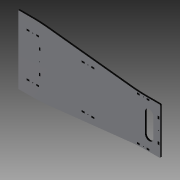
# Autodesk Inventor part: SIDE PLATE
Saved by Autodesk Inventor 2013 (Build 170138000, 138)
## iProperties
Created: 2014-06-21
Part Number: SIDE PLATE
Material: Generic
Document SubType Name: Modeling
Designer: employee
Density: 1 g/cm^3
Author: employee
Autodesk Inventor part; units mm, degrees
ref_plane "YZ Plane" through (0, 0, 0) normal (1, 0, 0) x (0, 1, 0)
ref_plane "XZ Plane" through (0, 0, 0) normal (0, 1, 0) x (-1, 0, 0)
ref_plane "XY Plane" through (0, 0, 0) normal (0, 0, 1) x (1, 0, 0)
sketch "Sketch1" plane through (0, 0, 0) normal (0, 0, 1) x (1, 0, 0)
  line L0 (508.715, -158.715) -> (-5.715, -158.715) construction
  line L1 (-5.715, -158.715) -> (-5.715, 8.715)
  line L2 (-5.715, 8.715) -> (508.715, 8.715) construction
  line L3 (508.715, 8.715) -> (508.715, -158.715)
  line L4 (-5.715, 8.715) -> (-5.715, 48.715)
  line L5 (-5.715, 48.715) -> (44.285, 48.715)
  arc A0 (99.6722, 45.6378) -> (44.285, 48.715) centre (44.285, -451.285) ccw
  line L6 (99.6722, 45.6378) -> (403.3278, 11.7922)
  arc A1 (403.3278, 11.7922) -> (458.715, 8.715) centre (458.715, 508.715) ccw
  line L7 (458.715, 8.715) -> (508.715, 8.715)
  line L8 (-5.715, -158.715) -> (-5.715, -198.715)
  line L9 (-5.715, -198.715) -> (44.285, -198.715)
  arc A2 (44.285, -198.715) -> (99.6722, -195.6378) centre (44.285, 301.285) ccw
  line L10 (99.6722, -195.6378) -> (403.3278, -161.7922)
  arc A3 (458.715, -158.715) -> (403.3278, -161.7922) centre (458.715, -658.715) ccw
  line L11 (458.715, -158.715) -> (508.715, -158.715)
  point P0 (0, 0)
  point P1 (0, 5.715)
  point P2 (505.715, -158.715)
  point P3 (505.715, 8.715)
  point P4 (-5.715, 5.715)
  dimension "d0" = 3
  dimension "d2" = 500
  dimension "d3" = 50
  dimension "d4" = 40
  constraints: 24 end point, 8 point on circle, 8 tangent, 4 centre point, 4 equal length, 4 parallel, 4 perpendicular, 3 equal radius, 3 point on line, 2 horizontal, 4 other
  measures "d0" distance from line of L3 point (505.715, -158.715)
  measures "d2" radius of A0
  measures "d3" distance of L4.end L5.end
  measures "d4" distance of L0.end L8.end
extrude "Extrusion1" add sketch "Sketch1" along normal blind 5.715
fillet "Fillet1" radius 3 2 edges at (508.715, 8.715, 2.8575) (508.715, -158.715, 2.8575)
sketch "Sketch2" plane through (0, 0, 5.715) normal (0, 0, 1) x (1, 0, 0)
  line L0 (24.6425, 0) -> (34.6425, 0) projected
  line L1 (34.6425, 5.715) -> (34.6425, 0) projected
  line L2 (34.6425, 5.715) -> (24.6425, 5.715) projected
  line L3 (24.6425, 5.715) -> (24.6425, 0) projected
  line L4 (59.6425, 0) -> (69.6425, 0) projected
  line L5 (69.6425, 5.715) -> (69.6425, 0) projected
  line L6 (69.6425, 5.715) -> (59.6425, 5.715) projected
  line L7 (59.6425, 5.715) -> (59.6425, 0) projected
  line L8 (224.6425, 0) -> (234.6425, 0) projected
  line L9 (234.6425, 5.715) -> (234.6425, 0) projected
  line L10 (234.6425, 5.715) -> (224.6425, 5.715) projected
  line L11 (224.6425, 5.715) -> (224.6425, 0) projected
  line L12 (259.6425, 0) -> (269.6425, 0) projected
  line L13 (269.6425, 5.715) -> (269.6425, 0) projected
  line L14 (269.6425, 5.715) -> (259.6425, 5.715) projected
  line L15 (259.6425, 5.715) -> (259.6425, 0) projected
  line L16 (424.6425, 0) -> (434.6425, 0) projected
  line L17 (434.6425, 5.715) -> (434.6425, 0) projected
  line L18 (434.6425, 5.715) -> (424.6425, 5.715) projected
  line L19 (424.6425, 5.715) -> (424.6425, 0) projected
  line L20 (459.6425, 0) -> (469.6425, 0) projected
  line L21 (469.6425, 5.715) -> (469.6425, 0) projected
  line L22 (469.6425, 5.715) -> (459.6425, 5.715) projected
  line L23 (459.6425, 5.715) -> (459.6425, 0) projected
  line L24 (500, -40) -> (500, -30) projected
  line L25 (505.715, -40) -> (500, -40) projected
  line L26 (505.715, -30) -> (505.715, -40) projected
  line L27 (505.715, -30) -> (500, -30) projected
  line L28 (500, -120) -> (500, -110) projected
  line L29 (505.715, -120) -> (500, -120) projected
  line L30 (505.715, -110) -> (505.715, -120) projected
  line L31 (505.715, -110) -> (500, -110) projected
  line L32 (459.6425, -155.715) -> (469.6425, -155.715) projected
  line L33 (469.6425, -150) -> (469.6425, -155.715) projected
  line L34 (469.6425, -150) -> (459.6425, -150) projected
  line L35 (459.6425, -150) -> (459.6425, -155.715) projected
  line L36 (424.6425, -155.715) -> (434.6425, -155.715) projected
  line L37 (434.6425, -150) -> (434.6425, -155.715) projected
  line L38 (434.6425, -150) -> (424.6425, -150) projected
  line L39 (424.6425, -150) -> (424.6425, -155.715) projected
  line L40 (259.6425, -155.715) -> (269.6425, -155.715) projected
  line L41 (269.6425, -150) -> (269.6425, -155.715) projected
  line L42 (269.6425, -150) -> (259.6425, -150) projected
  line L43 (259.6425, -150) -> (259.6425, -155.715) projected
  line L44 (224.6425, -155.715) -> (234.6425, -155.715) projected
  line L45 (234.6425, -150) -> (234.6425, -155.715) projected
  line L46 (234.6425, -150) -> (224.6425, -150) projected
  line L47 (224.6425, -150) -> (224.6425, -155.715) projected
  line L48 (59.6425, -155.715) -> (69.6425, -155.715) projected
  line L49 (69.6425, -150) -> (69.6425, -155.715) projected
  line L50 (69.6425, -150) -> (59.6425, -150) projected
  line L51 (59.6425, -150) -> (59.6425, -155.715) projected
  line L52 (24.6425, -155.715) -> (34.6425, -155.715) projected
  line L53 (34.6425, -150) -> (34.6425, -155.715) projected
  line L54 (34.6425, -150) -> (24.6425, -150) projected
  line L55 (24.6425, -150) -> (24.6425, -155.715) projected
  line L56 (34.6425, 2.8575) -> (59.6425, 2.8575) construction
  circle A0 centre (47.1425, 2.8575) radius 1.5
  line L57 (234.6425, 2.8575) -> (259.6425, 2.8575) construction
  circle A1 centre (247.1425, 2.8575) radius 1.5
  line L58 (434.6425, 2.8575) -> (459.6425, 2.8575) construction
  circle A2 centre (447.1425, 2.8575) radius 1.5
  line L59 (502.8575, -40) -> (502.8575, -110) construction
  circle A3 centre (502.8575, -75) radius 1.5
  line L60 (434.6425, -152.8575) -> (459.6425, -152.8575) construction
  circle A4 centre (447.1425, -152.8575) radius 1.5
  line L61 (234.6425, -152.8575) -> (259.6425, -152.8575) construction
  circle A5 centre (247.1425, -152.8575) radius 1.5
  line L62 (34.6425, -152.8575) -> (59.6425, -152.8575) construction
  circle A6 centre (47.1425, -152.8575) radius 1.5
  point P0 (0, 0)
  dimension "d8" = 3
  dimension "d10" = 3
  dimension "d11" = 3
  dimension "d12" = 3
  dimension "d13" = 3
  dimension "d14" = 3
  dimension "d15" = 3
  constraints: 21 midpoint, 14 end point, 7 centre point, 2 parallel
  measures "d8" diameter of A0
  measures "d10" diameter of A1
  measures "d11" diameter of A2
  measures "d12" diameter of A3
  measures "d13" diameter of A4
  measures "d14" diameter of A5
  measures "d15" diameter of A6
extrude "Extrusion2" cut sketch "Sketch2" against normal through all
sketch "Sketch3" plane through (0, 0, 5.715) normal (0, 0, 1) x (1, 0, 0)
  line L0 (75, -30) -> (75, -40) projected
  line L1 (75, -30) -> (69.285, -30) projected
  line L2 (69.285, -40) -> (69.285, -30) projected
  line L3 (75, -40) -> (69.285, -40) projected
  line L4 (75, -110) -> (75, -120) projected
  line L5 (75, -110) -> (69.285, -110) projected
  line L6 (69.285, -120) -> (69.285, -110) projected
  line L7 (75, -120) -> (69.285, -120) projected
  line L8 (72.1425, -40) -> (72.1425, -110)
  circle A0 centre (72.1425, -75) radius 1.5
  point P0 (0, 0)
  dimension "d18" = 3
  constraints: 3 midpoint, 2 end point, 1 centre point
  measures "d18" diameter of A0
extrude "Extrusion3" cut sketch "Sketch3" against normal through all
sketch "Sketch4" plane through (0, 0, 5.715) normal (0, 0, 1) x (1, 0, 0)
  circle A0 centre (502.8575, -75) radius 1.5 projected
  line L0 (508.715, -155.715) -> (508.715, 5.715) projected
  line L1 (458.715, -158.715) -> (505.715, -158.715) projected
  line L2 (453.715, -110) -> (453.715, -40)
  arc A1 (483.715, -40) -> (453.715, -40) centre (468.715, -40) ccw
  line L3 (483.715, -40) -> (483.715, -110)
  arc A2 (453.715, -110) -> (483.715, -110) centre (468.715, -110) ccw
  point P0 (0, 0)
  point P1 (483.715, -75)
  dimension "d22" = 70
  dimension "d25" = 15
  dimension "d26" = 25
  constraints: 4 end point, 4 point on circle, 4 tangent, 2 centre point, 1 horizontal alignment, 1 midpoint, 1 parallel, 1 perpendicular
  measures "d22" distance of L2.start L2.end
  measures "d25" radius of A1
  measures "d26" distance between parallel lines of L0 L3
extrude "Extrusion4" cut sketch "Sketch4" against normal through all contours L2 A1 L3 A2
body "Solid1"
